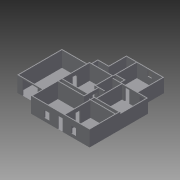
# Autodesk Inventor part: 286 College
Saved by Autodesk Inventor 2013 SP2 (Build 170200200, 200)
## iProperties
Created: 2014-06-02
Part Number: 286 College
Material: Generic
Document SubType Name: Modeling
Designer: jmw3
Density: 1 g/cm^3
Author: jmw3
Autodesk Inventor part; units mm, degrees
ref_plane "YZ Plane" through (0, 0, 0) normal (1, 0, 0) x (0, 1, 0)
ref_plane "XZ Plane" through (0, 0, 0) normal (0, 1, 0) x (-1, 0, 0)
ref_plane "XY Plane" through (0, 0, 0) normal (0, 0, 1) x (1, 0, 0)
sketch "Sketch1" plane through (0, 0, 0) normal (0, 1, 0) x (-1, 0, 0)
  line L0 (4978.4, 4978.4) -> (4978.4, -4978.4)
  line L1 (7823.2, 0) -> (-12090.4, 0) projected
  line L2 (0, -7853.68) -> (0, 12273.28) projected
  line L3 (3302, 4978.4) -> (3302, 9398)
  line L4 (3302, 9398) -> (-3124.2, 9398)
  line L5 (-9245.6, 4546.6) -> (-4978.4, 4546.6)
  line L6 (-9245.6, -3073.4) -> (-9245.6, 4546.6)
  line L7 (-4826, 4978.4) -> (-3098.8, 4978.4)
  line L8 (3302, 4978.4) -> (4978.4, 4978.4)
  line L9 (3149.6, 9245.6) -> (3149.6, 4978.4)
  line L10 (-2971.8, 6248.4) -> (-2971.8, 9245.6)
  line L11 (-1346.2, 4978.4) -> (-1346.2, 9245.6)
  line L12 (-4826, 4978.4) -> (-3098.8, 4978.4)
  line L13 (-3124.2, 6400.8) -> (-4978.4, 6400.8)
  line L14 (-4826, 4978.4) -> (-4826, 6248.4)
  line L15 (-3124.2, 9398) -> (-3124.2, 6400.8)
  line L16 (-4826, 6248.4) -> (-2971.8, 6248.4)
  line L17 (-4978.4, 6400.8) -> (-4978.4, 4546.6)
  line L18 (-3098.8, 4978.4) -> (-2946.4, 4978.4)
  line L19 (406.4, -4826) -> (406.4, -4978.4)
  line L20 (-406.4, -4826) -> (-406.4, -4978.4)
  line L21 (-4978.4, 4394.2) -> (-9093.2, 4394.2)
  line L22 (-9093.2, 4394.2) -> (-9093.2, -2921)
  line L23 (-8331.2, -2921) -> (-8331.2, -3073.4)
  line L24 (-5740.4, -2921) -> (-5740.4, -3073.4)
  line L25 (-4978.4, -3073.4) -> (-5740.4, -3073.4)
  line L26 (-8331.2, -3073.4) -> (-9245.6, -3073.4)
  line L27 (-9093.2, -2921) -> (-8331.2, -2921)
  line L28 (-5740.4, -2921) -> (-4978.4, -2921)
  line L29 (-406.4, -4826) -> (-4826, -4826)
  line L30 (4978.4, -4978.4) -> (406.4, -4978.4)
  line L31 (-406.4, -4978.4) -> (-4978.4, -4978.4)
  line L32 (-4978.4, -4978.4) -> (-4978.4, -3073.4)
  line L33 (-4978.4, 4546.6) -> (-4978.4, 4978.4)
  line L34 (4826, -4826) -> (711.2, -4826)
  line L35 (558.8, -4826) -> (406.4, -4826)
  line L36 (-4826, -406.4) -> (-533.4, -406.4)
  line L37 (711.2, -406.4) -> (4826, -406.4)
  line L38 (4826, -558.8) -> (711.2, -558.8)
  line L39 (-381, 889) -> (-533.4, 889)
  line L40 (558.8, 1930.4) -> (-381, 1930.4)
  line L41 (-600.7082, 2082.8) -> (558.8, 2082.8)
  line L42 (-533.4, 1752.6) -> (-381, 1752.6)
  line L43 (-381, 1752.6) -> (-381, 1930.4)
  line L44 (-600.7082, 2082.8) -> (-685.8, 2082.8)
  line L45 (-533.4, 1930.4) -> (-533.4, 1752.6)
  line L46 (558.8, 1143) -> (711.2, 1143)
  line L47 (558.8, 355.6) -> (711.2, 355.6)
  line L48 (711.2, 4826) -> (711.2, 1143)
  line L49 (558.8, -406.4) -> (558.8, 355.6)
  line L50 (558.8, 1143) -> (558.8, 1930.4)
  line L51 (558.8, 2082.8) -> (558.8, 4826)
  line L52 (-939.8, 2082.8) -> (-685.8, 2082.8)
  line L53 (-533.4, 1930.4) -> (-1092.2, 1930.4)
  line L54 (-1092.2, 1930.4) -> (-1092.2, 1930.4)
  line L55 (-939.8, 2082.8) -> (-939.8, 4826)
  line L56 (-1092.2, 4826) -> (-1092.2, 1930.4)
  line L57 (-381, -558.8) -> (-4826, -558.8)
  line L58 (558.8, -406.4) -> (406.4, -406.4)
  line L59 (406.4, -406.4) -> (406.4, -558.8)
  line L60 (406.4, -558.8) -> (558.8, -558.8)
  line L61 (-4826, -4826) -> (-4826, -558.8)
  line L62 (-4826, 254) -> (-533.4, 254)
  line L63 (-533.4, 101.6) -> (-4826, 101.6)
  line L64 (-533.4, 889) -> (-533.4, 254)
  line L65 (-533.4, 101.6) -> (-533.4, -406.4)
  line L66 (-4826, -406.4) -> (-4826, 101.6)
  line L67 (-319.4156, 5740.4) -> (406.4, 5740.4)
  line L68 (406.4, 5740.4) -> (406.4, 4978.4)
  line L69 (-1193.8, 5740.4) -> (406.4, 5740.4)
  line L70 (1955.8, 4978.4) -> (1955.8, 4826)
  line L71 (1168.4, 4978.4) -> (1168.4, 4826)
  line L72 (3149.6, 4978.4) -> (1955.8, 4978.4)
  line L73 (1955.8, 4826) -> (4826, 4826)
  line L74 (-1346.2, 4978.4) -> (-2946.4, 4978.4)
  line L75 (-4826, 4826) -> (-1092.2, 4826)
  line L76 (-939.8, 4826) -> (558.8, 4826)
  line L77 (711.2, 4826) -> (1168.4, 4826)
  line L78 (711.2, 254) -> (4826, 254)
  line L79 (4826, 101.6) -> (711.2, 101.6)
  line L80 (711.2, 355.6) -> (711.2, 254)
  line L81 (711.2, 101.6) -> (711.2, -406.4)
  line L82 (4826, 4826) -> (4826, 254)
  line L83 (4826, 101.6) -> (4826, -406.4)
  line L84 (4826, -558.8) -> (4826, -4826)
  line L85 (-381, 889) -> (-381, -558.8)
  line L86 (-4978.4, 1930.4) -> (-4826, 1930.4)
  line L87 (-4978.4, 2768.6) -> (-4826, 2768.6)
  line L88 (-4826, 254) -> (-4826, 1930.4)
  line L89 (-4826, 2768.6) -> (-4826, 4826)
  line L90 (-4978.4, 4394.2) -> (-4978.4, 2768.6)
  line L91 (-4978.4, 1930.4) -> (-4978.4, -2921)
  line L92 (-4978.4, -2921) -> (-4978.4, 1930.4)
  line L93 (-4978.4, 2768.6) -> (-4978.4, 4394.2)
  line L94 (-4978.4, -2921) -> (-4978.4, 1930.4)
  line L95 (-4978.4, 2768.6) -> (-4978.4, 4394.2)
  line L96 (558.8, -3073.4) -> (711.2, -3073.4)
  line L97 (558.8, -2286) -> (711.2, -2286)
  line L98 (558.8, -4826) -> (558.8, -3073.4)
  line L99 (558.8, -2286) -> (558.8, -558.8)
  line L100 (711.2, -558.8) -> (711.2, -2286)
  line L101 (711.2, -3073.4) -> (711.2, -4826)
  line L102 (-533.4, 1930.4) -> (-1092.2, 1930.4)
  line L103 (-1092.2, 1930.4) -> (-1092.2, 4826)
  line L104 (-4978.4, 2768.6) -> (-4978.4, 4394.2)
  line L105 (-4978.4, 2768.6) -> (-4826, 2768.6)
  line L106 (-9245.6, 4546.6) -> (-4978.4, 4546.6)
  line L107 (-4978.4, 4546.6) -> (-4978.4, 6400.8)
  line L108 (-4978.4, 6400.8) -> (-3124.2, 6400.8)
  line L109 (-3124.2, 6400.8) -> (-3124.2, 9398)
  line L110 (-3124.2, 9398) -> (3302, 9398)
  line L111 (-2971.8, 9245.6) -> (-1346.2, 9245.6)
  line L112 (-1193.8, 9245.6) -> (3149.6, 9245.6)
  line L113 (1168.4, 4978.4) -> (406.4, 4978.4)
  line L114 (-1193.8, 9245.6) -> (-1193.8, 5740.4)
  line L115 (-9245.6, 4546.6) -> (-4978.4, 4546.6)
  line L116 (-4978.4, 6400.8) -> (-4978.4, 4546.6)
  line L117 (-4978.4, 4394.2) -> (-9093.2, 4394.2)
  line L118 (-4978.4, 4394.2) -> (-4978.4, 2768.6)
  line L119 (-1193.8, 5588) -> (254, 5588)
  line L120 (254, 5588) -> (254, 4978.4)
  line L121 (254, 4978.4) -> (-1193.8, 4978.4)
  line L122 (-1193.8, 4978.4) -> (-1193.8, 5588)
  line L123 (-9093.2, 4394.2) -> (-4978.4, 4394.2)
  line L124 (-9093.2, -2921) -> (-9093.2, 4394.2)
  line L125 (-4978.4, -2921) -> (-5740.4, -2921)
  line L126 (-8331.2, -2921) -> (-9093.2, -2921)
  line L127 (-4978.4, 4394.2) -> (-4978.4, 2768.6)
  line L128 (-4978.4, 1930.4) -> (-4978.4, -2921)
  line L129 (-1193.8, 9245.6) -> (3149.6, 9245.6)
  line L130 (3149.6, 9245.6) -> (3149.6, 5740.4)
  line L131 (406.4, 5740.4) -> (-1193.8, 5740.4)
  line L132 (-1193.8, 5740.4) -> (-1193.8, 9245.6)
  line L133 (4826, 4826) -> (4826, 254)
  line L134 (4826, 254) -> (711.2, 254)
  line L135 (711.2, 4826) -> (1168.4, 4826)
  line L136 (1955.8, 4826) -> (4826, 4826)
  line L137 (711.2, 254) -> (711.2, 355.6)
  line L138 (711.2, 1143) -> (711.2, 4826)
  line L139 (-939.8, 4826) -> (558.8, 4826)
  line L140 (558.8, 4826) -> (558.8, 2082.8)
  line L141 (558.8, 2082.8) -> (-939.8, 2082.8)
  line L142 (-939.8, 2082.8) -> (-939.8, 4826)
  point P0 (0, 0)
  dimension "d3" = 1676.4
  dimension "d16" = 152.4
  dimension "d20" = 1854.2
  dimension "d21" = 6426.2
  dimension "d22" = 152.4
  dimension "d23" = 152.4
  dimension "d24" = 4419.6
  dimension "d25" = 4572
  dimension "d27" = 152.4
  dimension "d28" = 152.4
  dimension "d31" = 914.4
  dimension "d32" = 3505.2
  dimension "d33" = 152.4
  dimension "d34" = 7620
  dimension "d38" = 9956.8
  dimension "d40" = 1905
  dimension "d41" = 9956.8
  dimension "d43" = 152.4
  dimension "d46" = 152.4
  dimension "d47" = 4267.2
  dimension "d50" = 152.4
  dimension "d60" = 152.4
  dimension "d62" = 152.4
  dimension "d65" = 152.4
  dimension "d66" = 152.4
  dimension "d67" = 152.4
  dimension "d73" = 152.4
  dimension "d76" = 558.8
  dimension "d86" = 152.4
  dimension "d88" = 4267.2
  dimension "d89" = 863.6
  dimension "d90" = 787.4
  dimension "d92" = 2895.6
  dimension "d93" = 4470.4
  dimension "d94" = 152.4
  dimension "d95" = 4572
  dimension "d96" = 4572
  dimension "d97" = 4114.8
  dimension "d98" = 787.4
  dimension "d100" = 152.4
  dimension "d101" = 4445
  dimension "d103" = 1676.4
  dimension "d104" = 2514.6
  dimension "d105" = 4267.2
  dimension "d106" = 152.4
  dimension "d107" = 1854.2
  dimension "d108" = 1752.6
  dimension "d109" = 2540
  dimension "d111" = 5384.8
  dimension "d112" = 3657.6
  dimension "d113" = 635
  dimension "d114" = 152.4
  dimension "d115" = 3505.2
  dimension "d116" = 152.4
  dimension "d117" = 4343.4
  dimension "d119" = 152.4
  dimension "d120" = 152.4
  dimension "d121" = 152.4
  dimension "d122" = 2743.2
  dimension "d161" = 812.8
  constraints: 282 end point, 101 parallel, 68 perpendicular, 53 collinear, 25 horizontal, 2 point on line, 2 other
  measures "d3" distance between parallel lines of L0 L3
  measures "d16" distance between parallel lines of L3 L9
  measures "d20" distance between parallel lines of L13 L5
  measures "d21" distance between parallel lines of L3 L15
  measures "d22" distance between parallel lines of L15 L10
  measures "d23" distance between parallel lines of L13 L16
  measures "d24" distance between parallel lines of L8 L4
  measures "d25" distance between parallel lines of L0 L19
  measures "d27" distance between parallel lines of L6 L22
  measures "d28" distance between parallel lines of L5 L21
  measures "d31" distance between parallel lines of L6 L23
  measures "d32" distance between parallel lines of L6 L24
  measures "d33" distance between parallel lines of L26 L27
  measures "d34" distance between parallel lines of L26 L5
  measures "d38" distance between parallel lines of L30 L8
  measures "d40" distance between parallel lines of L31 L25
  measures "d41" distance between parallel lines of L0 L32
  measures "d43" distance between parallel lines of L31 L29
  measures "d46" distance between parallel lines of L38 L37
  measures "d47" distance between parallel lines of L34 L38
  measures "d50" distance between parallel lines of L40 L41
  measures "d60" distance between parallel lines of L48 L50
  measures "d62" distance between parallel lines of L52 L53
  measures "d65" distance between parallel lines of L56 L55
  measures "d66" distance of L49.start L58.end
  measures "d67" distance between parallel lines of L57 L36
  measures "d73" distance between parallel lines of L62 L63
  measures "d76" distance between parallel lines of L56 L45
  measures "d86" distance between parallel lines of L73 L8
  measures "d88" distance between parallel lines of L29 L57
  measures "d89" distance between parallel lines of L39 L42
  measures "d90" distance between parallel lines of L46 L47
  measures "d92" distance between parallel lines of L53 L75
  measures "d93" distance between parallel lines of L47 L77
  measures "d94" distance between parallel lines of L78 L79
  measures "d95" distance between parallel lines of L78 L73
  measures "d96" distance between parallel lines of L75 L62
  measures "d97" distance between parallel lines of L82 L48
  measures "d98" distance between parallel lines of L70 L71
  measures "d100" distance between parallel lines of L65 L85
  measures "d101" distance between parallel lines of L61 L85
  measures "d103" distance between parallel lines of L62 L86
  measures "d104" distance between parallel lines of L62 L87
  measures "d105" distance between parallel lines of L17 L6
  measures "d106" distance between parallel lines of L93 L89
  measures "d107" distance between parallel lines of L17 L15
  measures "d108" distance between parallel lines of L34 L96
  measures "d109" distance between parallel lines of L34 L97
  measures "d111" distance between parallel lines of L61 L99
  measures "d112" distance between parallel lines of L82 L71
  measures "d113" distance between parallel lines of L62 L39
  measures "d114" distance between parallel lines of L4 L111
  measures "d115" distance between parallel lines of L67 L112
  measures "d116" distance between parallel lines of L11 L114
  measures "d117" distance between parallel lines of L9 L114
  measures "d119" distance between parallel lines of L76 L121
  measures "d120" distance between parallel lines of L69 L119
  measures "d121" distance between parallel lines of L68 L120
  measures "d122" distance between parallel lines of L9 L68
  measures "d161" distance between parallel lines of L19 L20
extrude "Extrusion1" add sketch "Sketch1" along normal blind 2286 contours L0 L1 L83 L79 L81 L49 L47 L80 L78 L82 L73 L70 L72 L9 L112 L2 L4 L3 L8 | L0 L30 L19 L35 L98 L96 L101 L34 L84 L38 L100 L97 L99 L60 L59 L58 L49 L1 L81 L37 L83 | L2 L112 L114 L69 L67 L119 L122 L121 L76 L55 L52 L44 L41 L40 L43 L42 L45 L53 L56 L75 L89 L87 L90 L21 L22 L1 L6 L5 L17 L13 L15 L4 | L67 L68 L113 L71 L77 L48 L46 L50 L40 L2 L41 L51 L76 L121 L120 L119 | L85 L57 L61 L29 L20 L31 L32 L25 L24 L28 L91 L1 L66 L36 L65 | L1 L65 L63 L66 L91 L86 L88 L62 L64 L39 L85 | L22 L27 L23 L26 L6 L1
sketch "Sketch2" plane through (0, 0, 0) normal (0, -1, 0) x (1, 0, 0)
  line L0 (1346.2, 9245.6) -> (2971.8, 9245.6) projected
  line L1 (2971.8, 9245.6) -> (2971.8, 6248.4) projected
  line L2 (2971.8, 6248.4) -> (4826, 6248.4) projected
  line L3 (4826, 6248.4) -> (4826, 4978.4) projected
  line L4 (4826, 4978.4) -> (1346.2, 4978.4) projected
  line L5 (1346.2, 4978.4) -> (1346.2, 9245.6) projected
  line L6 (-558.8, 4826) -> (939.8, 4826) projected
  line L7 (939.8, 4826) -> (939.8, 2082.8) projected
  line L8 (939.8, 2082.8) -> (-558.8, 2082.8) projected
  line L9 (-558.8, 2082.8) -> (-558.8, 4826) projected
  line L10 (-711.2, 101.6) -> (-711.2, -406.4) projected
  line L11 (-711.2, -406.4) -> (-4826, -406.4) projected
  line L12 (-4826, -406.4) -> (-4826, 101.6) projected
  line L13 (-4826, 101.6) -> (-711.2, 101.6) projected
  line L14 (-254, 4978.4) -> (-254, 5588) projected
  line L15 (-254, 5588) -> (1193.8, 5588) projected
  line L16 (1193.8, 5588) -> (1193.8, 4978.4) projected
  line L17 (1193.8, 4978.4) -> (-254, 4978.4) projected
  line L18 (-4978.4, -4978.4) -> (-4978.4, 4978.4) projected
  line L19 (-406.4, -4978.4) -> (-4978.4, -4978.4) projected
  line L20 (-406.4, -4826) -> (-406.4, -4978.4) projected
  line L21 (-558.8, -4826) -> (-406.4, -4826) projected
  line L22 (-558.8, -3073.4) -> (-558.8, -4826) projected
  line L23 (-711.2, -3073.4) -> (-558.8, -3073.4) projected
  line L24 (-711.2, -4826) -> (-711.2, -3073.4) projected
  line L25 (-4826, -4826) -> (-711.2, -4826) projected
  line L26 (-4826, -558.8) -> (-4826, -4826) projected
  line L27 (-711.2, -558.8) -> (-4826, -558.8) projected
  line L28 (-711.2, -2286) -> (-711.2, -558.8) projected
  line L29 (-558.8, -2286) -> (-711.2, -2286) projected
  line L30 (-558.8, -558.8) -> (-558.8, -2286) projected
  line L31 (-406.4, -558.8) -> (-558.8, -558.8) projected
  line L32 (-406.4, -406.4) -> (-406.4, -558.8) projected
  line L33 (-558.8, -406.4) -> (-406.4, -406.4) projected
  line L34 (-558.8, 355.6) -> (-558.8, -406.4) projected
  line L35 (-711.2, 355.6) -> (-558.8, 355.6) projected
  line L36 (-711.2, 254) -> (-711.2, 355.6) projected
  line L37 (-4826, 254) -> (-711.2, 254) projected
  line L38 (-4826, 4826) -> (-4826, 254) projected
  line L39 (-1955.8, 4826) -> (-4826, 4826) projected
  line L40 (-1955.8, 4978.4) -> (-1955.8, 4826) projected
  line L41 (-3149.6, 4978.4) -> (-1955.8, 4978.4) projected
  line L42 (-3149.6, 9245.6) -> (-3149.6, 4978.4) projected
  line L43 (1193.8, 9245.6) -> (-3149.6, 9245.6) projected
  line L44 (1193.8, 5740.4) -> (1193.8, 9245.6) projected
  line L45 (-406.4, 5740.4) -> (1193.8, 5740.4) projected
  line L46 (-406.4, 4978.4) -> (-406.4, 5740.4) projected
  line L47 (-1168.4, 4978.4) -> (-406.4, 4978.4) projected
  line L48 (-1168.4, 4826) -> (-1168.4, 4978.4) projected
  line L49 (-711.2, 4826) -> (-1168.4, 4826) projected
  line L50 (-711.2, 1143) -> (-711.2, 4826) projected
  line L51 (-558.8, 1143) -> (-711.2, 1143) projected
  line L52 (-558.8, 1930.4) -> (-558.8, 1143) projected
  line L53 (381, 1930.4) -> (-558.8, 1930.4) projected
  line L54 (381, 1752.6) -> (381, 1930.4) projected
  line L55 (533.4, 1752.6) -> (381, 1752.6) projected
  line L56 (533.4, 1930.4) -> (533.4, 1752.6) projected
  line L57 (1092.2, 1930.4) -> (533.4, 1930.4) projected
  line L58 (1092.2, 4826) -> (1092.2, 1930.4) projected
  line L59 (4826, 4826) -> (1092.2, 4826) projected
  line L60 (4826, 2768.6) -> (4826, 4826) projected
  line L61 (4978.4, 2768.6) -> (4826, 2768.6) projected
  line L62 (4978.4, 4394.2) -> (4978.4, 2768.6) projected
  line L63 (9093.2, 4394.2) -> (4978.4, 4394.2) projected
  line L64 (9093.2, -2921) -> (9093.2, 4394.2) projected
  line L65 (8331.2, -2921) -> (9093.2, -2921) projected
  line L66 (8331.2, -3073.4) -> (8331.2, -2921) projected
  line L67 (9245.6, -3073.4) -> (8331.2, -3073.4) projected
  line L68 (4978.4, 6400.8) -> (4978.4, 4546.6) projected
  line L69 (3124.2, 6400.8) -> (4978.4, 6400.8) projected
  line L70 (3124.2, 9398) -> (3124.2, 6400.8) projected
  line L71 (-4978.4, 4978.4) -> (-3302, 4978.4) projected
  line L72 (4826, 101.6) -> (4826, -406.4) projected
  line L73 (4826, -406.4) -> (533.4, -406.4) projected
  line L74 (533.4, -406.4) -> (533.4, 101.6) projected
  line L75 (533.4, 101.6) -> (4826, 101.6) projected
  line L76 (4978.4, -4978.4) -> (406.4, -4978.4) projected
  line L77 (4978.4, -3073.4) -> (4978.4, -4978.4) projected
  line L78 (5740.4, -3073.4) -> (4978.4, -3073.4) projected
  line L79 (5740.4, -2921) -> (5740.4, -3073.4) projected
  line L80 (4978.4, -2921) -> (5740.4, -2921) projected
  line L81 (4978.4, 1930.4) -> (4978.4, -2921) projected
  line L82 (4826, 1930.4) -> (4978.4, 1930.4) projected
  line L83 (4826, 254) -> (4826, 1930.4) projected
  line L84 (533.4, 254) -> (4826, 254) projected
  line L85 (533.4, 889) -> (533.4, 254) projected
  line L86 (381, 889) -> (533.4, 889) projected
  line L87 (381, -558.8) -> (381, 889) projected
  line L88 (4826, -558.8) -> (381, -558.8) projected
  line L89 (4826, -4826) -> (4826, -558.8) projected
  line L90 (406.4, -4826) -> (4826, -4826) projected
  line L91 (406.4, -4978.4) -> (406.4, -4826) projected
  line L92 (-4978.4, 4978.4) -> (4978.4, 4978.4)
  line L93 (4978.4, 4978.4) -> (4978.4, -4978.4)
  line L94 (4978.4, -4978.4) -> (-4978.4, -4978.4)
  line L95 (-4978.4, -4978.4) -> (-4978.4, 4978.4)
  line L96 (4978.4, 4546.6) -> (9245.6, 4546.6)
  line L97 (9245.6, 4546.6) -> (9245.6, -3073.4)
  line L98 (9245.6, -3073.4) -> (4978.4, -3073.4)
  line L99 (4978.4, -3073.4) -> (4978.4, 4546.6)
  line L100 (4978.4, 4978.4) -> (3124.2, 4978.4)
  line L101 (3124.2, 4978.4) -> (3124.2, 6400.8)
  line L102 (3124.2, 6400.8) -> (4978.4, 6400.8)
  line L103 (4978.4, 6400.8) -> (4978.4, 4978.4)
  line L104 (3124.2, 9398) -> (-3302, 9398)
  line L105 (-3302, 9398) -> (-3302, 4978.4)
  line L106 (-3302, 4978.4) -> (3124.2, 4978.4)
  line L107 (3124.2, 4978.4) -> (3124.2, 9398)
  point P0 (0, 0)
  constraints: 32 end point, 8 parallel, 4 horizontal, 4 perpendicular
extrude "Extrusion2" add sketch "Sketch2" along normal blind 25.4 contours L5 L92 L16 L15 L14 L46 L45 L44 L43 L42 L105 L104 L70 L101 L2 L1 L0 | L0 L1 L2 L101 L4 L5 | L4 L92 L68 L93 L62 L61 L60 L59 L58 L57 L56 L55 L54 L53 L52 L51 L50 L49 L48 L47 L17 | L101 L2 L3 L4 | L17 L14 L15 L16 | L101 L69 L68 L92 L3 L2 | L47 L92 L41 L42 L43 L44 L45 L46 | L96 L97 L67 L66 L65 L64 L63 L93 | L48 L49 L50 L51 L52 L53 L54 L55 L56 L57 L58 L59 L60 L61 L93 L82 L83 L84 L85 L86 L87 L88 L89 L90 L91 L94 L20 L21 L22 L23 L24 L25 L26 L27 L28 L29 L30 L31 L32 L33 L34 L35 L36 L37 L38 L39 L40 L92 | L63 L64 L65 L66 L98 L79 L80 L81 L93 L62 | L40 L39 L38 L37 L36 L35 L34 L33 L32 L31 L30 L29 L28 L27 L26 L25 L24 L23 L22 L21 L20 L19 L18 L71 L92 L41 | L81 L93 L77 L76 L91 L90 L89 L88 L87 L86 L85 L84 L83 L82 | L80 L79 L78 L93 | L6 L7 L8 L9 | L10 L11 L12 L13 | L72 L73 L74 L75
sketch "Sketch3" plane through (-406.4, 2286, -4978.4) normal (0, 0, -1) x (-1, 0, 0)
  line L0 (4572, 0) -> (4572, -2311.4) projected
  line L1 (0, 0) -> (4572, 0) projected
  line L2 (-5384.8, 0) -> (-812.8, 0) projected
  line L3 (-5384.8, 0) -> (-5384.8, -2311.4) projected
  line L4 (-812.8, -2286) -> (-5232.4, -2286) projected
  line L5 (152.4, -2286) -> (0, -2286) projected
  line L6 (4419.6, -2286) -> (304.8, -2286) projected
  line L7 (304.8, -2286) -> (152.4, -2286) projected
  line L8 (-3098.8, -635) -> (-2286, -635)
  line L9 (-2286, -635) -> (-2286, -1778)
  line L10 (-2286, -1778) -> (-3098.8, -1778)
  line L11 (-3098.8, -1778) -> (-3098.8, -635)
  line L12 (1473.2, -635) -> (2286, -635)
  line L13 (2286, -635) -> (2286, -1778)
  line L14 (2286, -1778) -> (1473.2, -1778)
  line L15 (1473.2, -1778) -> (1473.2, -635)
  point P0 (-406.4, -2286)
  dimension "d127" = 635
  dimension "d128" = 508
  dimension "d129" = 635
  dimension "d130" = 508
  dimension "d131" = 2286
  dimension "d132" = 3098.8
  dimension "d133" = 2286
  dimension "d134" = 3098.8
  constraints: 16 end point, 4 parallel, 2 horizontal, 2 perpendicular
  measures "d127" distance between parallel lines of L2 L8
  measures "d128" distance between parallel lines of L4 L10
  measures "d129" distance between parallel lines of L1 L12
  measures "d130" distance between parallel lines of L6 L14
  measures "d131" distance between parallel lines of L0 L13
  measures "d132" distance between parallel lines of L0 L15
  measures "d133" distance between parallel lines of L3 L11
  measures "d134" distance between parallel lines of L3 L9
extrude "Extrusion3" cut sketch "Sketch3" against normal up to surface (152.4 mm away)
sketch "Sketch4" plane through (-4978.4, 2286, 4978.4) normal (0, 0, 1) x (1, 0, 0)
  line L0 (1676.4, -2311.4) -> (1676.4, 0) projected
  line L1 (0, 0) -> (1676.4, 0) projected
  line L2 (0, -2311.4) -> (0, 0) projected
  line L3 (558.8, -304.8) -> (1295.4, -304.8)
  line L4 (1295.4, -304.8) -> (1295.4, -1727.2)
  line L5 (1295.4, -1727.2) -> (558.8, -1727.2)
  line L6 (558.8, -1727.2) -> (558.8, -304.8)
  line L7 (3022.6, -2286) -> (152.4, -2286) projected
  point P0 (4978.4, -2286)
  dimension "d137" = 304.8
  dimension "d138" = 558.8
  dimension "d139" = 381
  dimension "d140" = 558.8
  constraints: 8 end point, 2 parallel, 1 horizontal, 1 perpendicular
  measures "d137" distance between parallel lines of L1 L3
  measures "d138" distance between parallel lines of L7 L5
  measures "d139" distance between parallel lines of L0 L4
  measures "d140" distance between parallel lines of L2 L6
extrude "Extrusion4" cut sketch "Sketch4" against normal up to surface (152.4 mm away)
sketch "Sketch5" plane through (-3302, 2286, 9398) normal (0, 0, 1) x (1, 0, 0)
  line L0 (0, 0) -> (6426.2, 0) projected
  line L1 (0, -2311.4) -> (0, 0) projected
  line L2 (6426.2, -2311.4) -> (0, -2311.4) projected
  line L3 (1981.2, -203.2) -> (2667, -203.2)
  line L4 (2667, -203.2) -> (2667, -1117.6)
  line L5 (2667, -1117.6) -> (1981.2, -1117.6)
  line L6 (1981.2, -1117.6) -> (1981.2, -203.2)
  point P0 (3302, -2286)
  dimension "d143" = 203.2
  dimension "d144" = 1193.8
  dimension "d145" = 1981.2
  dimension "d146" = 2667
  constraints: 8 end point, 2 parallel, 1 horizontal, 1 perpendicular
  measures "d143" distance between parallel lines of L0 L3
  measures "d144" distance between parallel lines of L2 L5
  measures "d145" distance between parallel lines of L1 L6
  measures "d146" distance between parallel lines of L1 L4
extrude "Extrusion5" cut sketch "Sketch5" against normal up to surface (152.4 mm away)
sketch "Sketch6" plane through (0, 2286, 0) normal (0, 1, 0) x (1, 0, 0)
  line L0 (4826, 406.4) -> (4826, -101.6) projected
  line L1 (4826, -101.6) -> (533.4, -101.6) projected
  line L2 (533.4, -101.6) -> (533.4, 406.4) projected
  line L3 (533.4, 406.4) -> (4826, 406.4) projected
  line L4 (4978.4, 4978.4) -> (406.4, 4978.4) projected
  line L5 (406.4, 4978.4) -> (406.4, 4826) projected
  line L6 (406.4, 4826) -> (4826, 4826) projected
  line L7 (4826, 4826) -> (4826, 558.8) projected
  line L8 (4826, 558.8) -> (381, 558.8) projected
  line L9 (381, 558.8) -> (381, -889) projected
  line L10 (381, -889) -> (533.4, -889) projected
  line L11 (533.4, -889) -> (533.4, -254) projected
  line L12 (533.4, -254) -> (4826, -254) projected
  line L13 (4826, -254) -> (4826, -1930.4) projected
  line L14 (4826, -1930.4) -> (4978.4, -1930.4) projected
  line L15 (4978.4, -1930.4) -> (4978.4, 2921) projected
  line L16 (4978.4, 2921) -> (5740.4, 2921) projected
  line L17 (5740.4, 2921) -> (5740.4, 3073.4) projected
  line L18 (5740.4, 3073.4) -> (4978.4, 3073.4) projected
  line L19 (4978.4, 3073.4) -> (4978.4, 4978.4) projected
  line L20 (406.4, 4826) -> (-406.4, 4826)
  line L21 (-406.4, 4826) -> (-406.4, 4978.4)
  line L22 (-406.4, 4978.4) -> (406.4, 4978.4)
  line L23 (406.4, 4978.4) -> (406.4, 4826)
  line L24 (-558.8, 2286) -> (-711.2, 2286)
  line L25 (-711.2, 2286) -> (-711.2, 3073.4)
  line L26 (-711.2, 3073.4) -> (-558.8, 3073.4)
  line L27 (-558.8, 3073.4) -> (-558.8, 2286)
  line L28 (-558.8, -1143) -> (-711.2, -1143)
  line L29 (-711.2, -1143) -> (-711.2, -355.6)
  line L30 (-711.2, -355.6) -> (-558.8, -355.6)
  line L31 (-558.8, -355.6) -> (-558.8, -1143)
  line L32 (533.4, -1752.6) -> (381, -1752.6)
  line L33 (381, -1752.6) -> (381, -889)
  line L34 (381, -889) -> (533.4, -889)
  line L35 (533.4, -889) -> (533.4, -1752.6)
  line L36 (-1168.4, -4978.4) -> (-1955.8, -4978.4)
  line L37 (-1955.8, -4978.4) -> (-1955.8, -4826)
  line L38 (-1955.8, -4826) -> (-1168.4, -4826)
  line L39 (-1168.4, -4826) -> (-1168.4, -4978.4)
  line L40 (4978.4, -2768.6) -> (4826, -2768.6)
  line L41 (4826, -2768.6) -> (4826, -1930.4)
  line L42 (4826, -1930.4) -> (4978.4, -1930.4)
  line L43 (4978.4, -1930.4) -> (4978.4, -2768.6)
  line L44 (2971.8, -9245.6) -> (1346.2, -9245.6) projected
  line L45 (1346.2, -9245.6) -> (1346.2, -4978.4) projected
  line L46 (1346.2, -4978.4) -> (4826, -4978.4) projected
  line L47 (4826, -4978.4) -> (4826, -6248.4) projected
  line L48 (4826, -6248.4) -> (2971.8, -6248.4) projected
  line L49 (2971.8, -6248.4) -> (2971.8, -9245.6) projected
  line L50 (939.8, -4826) -> (-558.8, -4826) projected
  line L51 (-558.8, -4826) -> (-558.8, -2082.8) projected
  line L52 (-558.8, -2082.8) -> (939.8, -2082.8) projected
  line L53 (939.8, -2082.8) -> (939.8, -4826) projected
  line L54 (-711.2, 406.4) -> (-711.2, -101.6) projected
  line L55 (-711.2, -101.6) -> (-4826, -101.6) projected
  line L56 (-4826, -101.6) -> (-4826, 406.4) projected
  line L57 (-4826, 406.4) -> (-711.2, 406.4) projected
  line L58 (-254, -5588) -> (-254, -4978.4) projected
  line L59 (-254, -4978.4) -> (1193.8, -4978.4) projected
  line L60 (1193.8, -4978.4) -> (1193.8, -5588) projected
  line L61 (1193.8, -5588) -> (-254, -5588) projected
  line L62 (-4978.4, 4978.4) -> (-4978.4, -4978.4) projected
  line L63 (-4978.4, -4978.4) -> (-3302, -4978.4) projected
  line L64 (-3302, -4978.4) -> (-3302, -9398) projected
  line L65 (-3302, -9398) -> (3124.2, -9398) projected
  line L66 (3124.2, -9398) -> (3124.2, -6400.8) projected
  line L67 (3124.2, -6400.8) -> (4978.4, -6400.8) projected
  line L68 (4978.4, -6400.8) -> (4978.4, -4546.6) projected
  line L69 (4978.4, -4546.6) -> (9245.6, -4546.6) projected
  line L70 (9245.6, -4546.6) -> (9245.6, 3073.4) projected
  line L71 (9245.6, 3073.4) -> (8331.2, 3073.4) projected
  line L72 (8331.2, 3073.4) -> (8331.2, 2921) projected
  line L73 (8331.2, 2921) -> (9093.2, 2921) projected
  line L74 (9093.2, 2921) -> (9093.2, -4394.2) projected
  line L75 (9093.2, -4394.2) -> (4978.4, -4394.2) projected
  line L76 (4978.4, -4394.2) -> (4978.4, -2768.6) projected
  line L77 (4978.4, -2768.6) -> (4826, -2768.6) projected
  line L78 (4826, -2768.6) -> (4826, -4826) projected
  line L79 (4826, -4826) -> (1092.2, -4826) projected
  line L80 (1092.2, -4826) -> (1092.2, -1930.4) projected
  line L81 (1092.2, -1930.4) -> (533.4, -1930.4) projected
  line L82 (533.4, -1930.4) -> (533.4, -1752.6) projected
  line L83 (533.4, -1752.6) -> (381, -1752.6) projected
  line L84 (381, -1752.6) -> (381, -1930.4) projected
  line L85 (381, -1930.4) -> (-558.8, -1930.4) projected
  line L86 (-558.8, -1930.4) -> (-558.8, -1143) projected
  line L87 (-558.8, -1143) -> (-711.2, -1143) projected
  line L88 (-711.2, -1143) -> (-711.2, -4826) projected
  line L89 (-711.2, -4826) -> (-1168.4, -4826) projected
  line L90 (-1168.4, -4826) -> (-1168.4, -4978.4) projected
  line L91 (-1168.4, -4978.4) -> (-406.4, -4978.4) projected
  line L92 (-406.4, -4978.4) -> (-406.4, -5740.4) projected
  line L93 (-406.4, -5740.4) -> (1193.8, -5740.4) projected
  line L94 (1193.8, -5740.4) -> (1193.8, -9245.6) projected
  line L95 (1193.8, -9245.6) -> (-3149.6, -9245.6) projected
  line L96 (-3149.6, -9245.6) -> (-3149.6, -4978.4) projected
  line L97 (-3149.6, -4978.4) -> (-1955.8, -4978.4) projected
  line L98 (-1955.8, -4978.4) -> (-1955.8, -4826) projected
  line L99 (-1955.8, -4826) -> (-4826, -4826) projected
  line L100 (-4826, -4826) -> (-4826, -254) projected
  line L101 (-4826, -254) -> (-711.2, -254) projected
  line L102 (-711.2, -254) -> (-711.2, -355.6) projected
  line L103 (-711.2, -355.6) -> (-558.8, -355.6) projected
  line L104 (-558.8, -355.6) -> (-558.8, 406.4) projected
  line L105 (-558.8, 406.4) -> (-406.4, 406.4) projected
  line L106 (-406.4, 406.4) -> (-406.4, 558.8) projected
  line L107 (-406.4, 558.8) -> (-558.8, 558.8) projected
  line L108 (-558.8, 558.8) -> (-558.8, 2286) projected
  line L109 (-558.8, 2286) -> (-711.2, 2286) projected
  line L110 (-711.2, 2286) -> (-711.2, 558.8) projected
  line L111 (-711.2, 558.8) -> (-4826, 558.8) projected
  line L112 (-4826, 558.8) -> (-4826, 4826) projected
  line L113 (-4826, 4826) -> (-711.2, 4826) projected
  line L114 (-711.2, 4826) -> (-711.2, 3073.4) projected
  line L115 (-711.2, 3073.4) -> (-558.8, 3073.4) projected
  line L116 (-558.8, 3073.4) -> (-558.8, 4826) projected
  line L117 (-558.8, 4826) -> (-406.4, 4826) projected
  line L118 (-406.4, 4826) -> (-406.4, 4978.4) projected
  line L119 (-406.4, 4978.4) -> (-4978.4, 4978.4) projected
  point P0 (0, 0)
  constraints: 48 end point, 12 parallel, 6 horizontal, 6 perpendicular
extrude "Extrusion6" add sketch "Sketch6" against normal blind 304.8 contours L5 L20 L21 L22 | L27 L24 L25 L26
extrude "Extrusion7" add sketch "Sketch6" against normal blind 279.4 contours L43 L40 L41 L14 | L28 L29 L30 L31
extrude "Extrusion8" add sketch "Sketch6" against normal blind 254 contours L39 L36 L37 L38
extrude "Extrusion9" add sketch "Sketch6" against normal blind 203.2 contours L10 L35 L32 L33
sketch "Sketch7" plane through (0, 2286, 0) normal (0, 1, 0) x (1, 0, 0)
  line L0 (381, 558.8) -> (381, -1930.4) projected
  line L1 (381, -1930.4) -> (-558.8, -1930.4) projected
  line L2 (-558.8, -1930.4) -> (-558.8, 406.4) projected
  line L3 (-558.8, 406.4) -> (-406.4, 406.4) projected
  line L4 (-406.4, 406.4) -> (-406.4, 558.8) projected
  line L5 (-406.4, 558.8) -> (-558.8, 558.8) projected
  line L6 (-558.8, 558.8) -> (-558.8, 4826) projected
  line L7 (-558.8, 4826) -> (4826, 4826) projected
  line L8 (4826, 4826) -> (4826, 558.8) projected
  line L9 (4826, 558.8) -> (381, 558.8) projected
  line L10 (533.4, -1930.4) -> (533.4, -254) projected
  line L11 (533.4, -254) -> (4826, -254) projected
  line L12 (4826, -254) -> (4826, -4826) projected
  line L13 (4826, -4826) -> (1092.2, -4826) projected
  line L14 (1092.2, -4826) -> (1092.2, -1930.4) projected
  line L15 (1092.2, -1930.4) -> (533.4, -1930.4) projected
  line L16 (4978.4, -4394.2) -> (4978.4, 2921) projected
  line L17 (4978.4, 2921) -> (5740.4, 2921) projected
  line L18 (5740.4, 2921) -> (5740.4, 3073.4) projected
  line L19 (5740.4, 3073.4) -> (4978.4, 3073.4) projected
  line L20 (4978.4, 3073.4) -> (4978.4, 4978.4) projected
  line L21 (4978.4, 4978.4) -> (-4978.4, 4978.4) projected
  line L22 (-4978.4, 4978.4) -> (-4978.4, -4978.4) projected
  line L23 (4978.4, -6400.8) -> (4978.4, -4546.6) projected
  line L24 (4978.4, -4546.6) -> (9245.6, -4546.6) projected
  line L25 (9245.6, -4546.6) -> (9245.6, 3073.4) projected
  line L26 (9245.6, 3073.4) -> (8331.2, 3073.4) projected
  line L27 (8331.2, 3073.4) -> (8331.2, 2921) projected
  line L28 (8331.2, 2921) -> (9093.2, 2921) projected
  line L29 (9093.2, 2921) -> (9093.2, -4394.2) projected
  line L30 (9093.2, -4394.2) -> (4978.4, -4394.2) projected
  line L31 (4826, 406.4) -> (4826, -101.6) projected
  line L32 (4826, -101.6) -> (533.4, -101.6) projected
  line L33 (533.4, -101.6) -> (533.4, 406.4) projected
  line L34 (533.4, 406.4) -> (4826, 406.4) projected
  line L35 (-711.2, 4826) -> (-711.2, 558.8) projected
  line L36 (-711.2, 558.8) -> (-4826, 558.8) projected
  line L37 (-4826, 558.8) -> (-4826, 4826) projected
  line L38 (-4826, 4826) -> (-711.2, 4826) projected
  line L39 (1346.2, -4978.4) -> (4826, -4978.4) projected
  line L40 (-558.8, -2082.8) -> (939.8, -2082.8) projected
  line L41 (939.8, -2082.8) -> (939.8, -4826) projected
  line L42 (-711.2, 406.4) -> (-711.2, -101.6) projected
  line L43 (-711.2, -101.6) -> (-4826, -101.6) projected
  line L44 (-4826, -101.6) -> (-4826, 406.4) projected
  line L45 (-4826, 406.4) -> (-711.2, 406.4) projected
  line L46 (-254, -4978.4) -> (1193.8, -4978.4) projected
  line L47 (-4826, -254) -> (-711.2, -254) projected
  line L48 (-711.2, -254) -> (-711.2, -4826) projected
  line L49 (-558.8, -2082.8) -> (-558.8, -1930.4)
  line L50 (1346.2, -4978.4) -> (1193.8, -4978.4)
  line L51 (939.8, -4826) -> (939.8, -4978.4)
  line L52 (4826, -4978.4) -> (4978.4, -4978.4)
  line L53 (-711.2, -254) -> (-558.8, -254)
  line L54 (-4826, -254) -> (-4978.4, -254)
  point P0 (0, 0)
  constraints: 12 end point, 4 perpendicular, 4 point on line, 2 parallel
extrude "Extrusion10" add sketch "Sketch7" along normal blind 330.2 contours L9 L8 L7 L6 L5 L4 L3 L2 L53 L47 L54 L22 L21 L20 L19 L18 L17 L16 L30 L29 L28 L27 L26 L25 L24 L23 L52 L39 L50 L46 L51 L41 L40 L49 L1 L0
sketch "Sketch8" plane through (0, 2616.2, 0) normal (0, 1, 0) x (1, 0, 0)
  line L0 (8331.2, 2921) -> (5740.4, 2921)
  line L1 (5740.4, 2921) -> (5740.4, 3073.4)
  line L2 (5740.4, 3073.4) -> (8331.2, 3073.4)
  line L3 (8331.2, 3073.4) -> (8331.2, 2921)
  line L4 (-406.4, 406.4) -> (381, 406.4)
  line L5 (381, 406.4) -> (381, 558.8)
  line L6 (381, 558.8) -> (-406.4, 558.8)
  line L7 (-406.4, 558.8) -> (-406.4, 406.4)
  point P0 (0, 0)
  constraints: 16 end point, 4 parallel, 2 horizontal, 2 perpendicular
extrude "Extrusion11" add sketch "Sketch8" against normal blind 203.2 contours L0 L1 L2 L3
body "Solid1"
